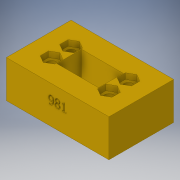
# Autodesk Inventor part: CapForCanBusConnector
Saved by Autodesk Inventor 2018.1 (Build 221171000, 171)
## iProperties
Created: 2017-10-25
Part Number: CapForCanBusConnector
Material: Generic
Document SubType Name: Modeling
Designer: steele
Density: 1 g/cm^3
Appearance: Gold
Author: steele
Autodesk Inventor part; units mm, degrees
note: some values were not read from the file. Chosen so that the rebuilt part matches the saved one: direction of "Emboss1".
ref_plane "YZ Plane" through (0, 0, 0) normal (1, 0, 0) x (0, 1, 0)
ref_plane "XZ Plane" through (0, 0, 0) normal (0, 1, 0) x (-1, 0, 0)
ref_plane "XY Plane" through (0, 0, 0) normal (0, 0, 1) x (1, 0, 0)
sketch "Sketch1" plane through (0, 0, 0) normal (0, 1, 0) x (-1, 0, 0)
  line L0 (18.6817, 11.7856) -> (-18.6817, 11.7856)
  line L1 (-18.6817, 11.7856) -> (-18.6817, -11.7856)
  line L2 (-18.6817, -11.7856) -> (18.6817, -11.7856)
  line L3 (18.6817, -11.7856) -> (18.6817, 11.7856)
  line L4 (18.6817, 11.7856) -> (-18.6817, -11.7856) construction
  line L5 (-18.6817, 11.7856) -> (18.6817, -11.7856) construction
  point P0 (0, 0)
  dimension "d0" = 37.3634
  dimension "d1" = 23.5712
  constraints: 12 end point, 2 midpoint, 2 parallel, 1 horizontal, 1 perpendicular
  measures "d0" distance of L1.end L2.end
  measures "d1" distance of L2.end L0.start
extrude "Extrusion1" add sketch "Sketch1" along normal blind 13.589
sketch "Sketch5" plane through (0, 0, 0) normal (0, -1, 0) x (1, 0, 0)
  line L0 (7.6073, 4.5085) -> (-7.6073, 4.5085)
  line L1 (-7.6073, 4.5085) -> (-7.6073, -4.5085)
  line L2 (-7.6073, -4.5085) -> (7.6073, -4.5085)
  line L3 (7.6073, -4.5085) -> (7.6073, 4.5085)
  line L4 (7.6073, 4.5085) -> (-7.6073, -4.5085) construction
  line L5 (-7.6073, 4.5085) -> (7.6073, -4.5085) construction
  point P0 (0, 0)
  dimension "d25" = 15.2146
  dimension "d26" = 9.017
  constraints: 12 end point, 2 midpoint, 2 parallel, 1 horizontal, 1 perpendicular
  measures "d25" distance of L1.end L2.end
  measures "d26" distance of L2.end L0.start
extrude "Extrusion3" cut sketch "Sketch5" against normal through all
sketch "Sketch8" plane through (0, 13.589, 0) normal (0, 1, 0) x (1, 0, 0)
  circle A0 centre (-10.4521, 3.556) radius 1.632 projected
  line L0 (-7.8168, 5.0775) -> (-7.8168, 2.0345)
  line L1 (-7.8168, 2.0345) -> (-10.4521, 0.5131)
  line L2 (-10.4521, 0.5131) -> (-13.0873, 2.0345)
  line L3 (-13.0873, 2.0345) -> (-13.0873, 5.0775)
  line L4 (-13.0873, 5.0775) -> (-10.4521, 6.5989)
  line L5 (-10.4521, 6.5989) -> (-7.8168, 5.0775)
  circle A1 centre (-10.4521, -3.556) radius 1.632 projected
  line L6 (-7.8169, -2.0345) -> (-7.8169, -5.0775)
  line L7 (-7.8169, -5.0775) -> (-10.4521, -6.5989)
  line L8 (-10.4521, -6.5989) -> (-13.0874, -5.0775)
  line L9 (-13.0874, -5.0775) -> (-13.0874, -2.0345)
  line L10 (-13.0874, -2.0345) -> (-10.4521, -0.5131)
  line L11 (-10.4521, -0.5131) -> (-7.8169, -2.0345)
  circle A2 centre (10.4521, -3.556) radius 1.632 projected
  line L12 (10.4521, -0.5131) -> (13.0873, -2.0345)
  line L13 (13.0873, -2.0345) -> (13.0873, -5.0775)
  line L14 (13.0873, -5.0775) -> (10.4521, -6.5989)
  line L15 (10.4521, -6.5989) -> (7.8168, -5.0775)
  line L16 (7.8168, -5.0775) -> (7.8168, -2.0345)
  line L17 (7.8168, -2.0345) -> (10.4521, -0.5131)
  circle A3 centre (10.4521, 3.556) radius 1.632 projected
  line L18 (13.0874, 5.0775) -> (13.0874, 2.0345)
  line L19 (13.0874, 2.0345) -> (10.4521, 0.5131)
  line L20 (10.4521, 0.5131) -> (7.8169, 2.0345)
  line L21 (7.8169, 2.0345) -> (7.8169, 5.0775)
  line L22 (7.8169, 5.0775) -> (10.4521, 6.5989)
  line L23 (10.4521, 6.5989) -> (13.0874, 5.0775)
  line L24 (18.6817, 11.7856) -> (-18.6817, 11.7856) construction
  line L25 (0, 11.7856) -> (0, -11.7856) construction
  line L26 (-18.6817, -11.7856) -> (18.6817, -11.7856) construction
  point P0 (0, 0)
  dimension "d43" = 5.2705
  constraints: 50 end point, 4 coincident, 4 parallel, 3 equal length, 2 midpoint, 52 other
  measures "d43" distance between parallel lines of L1 L4
extrude "Extrusion5" cut sketch "Sketch8" against normal blind 2.0955 contours A0 | L0 L1 L2 L3 L4 L5 | A1 | L6 L7 L8 L9 L10 L11 | A2 | L12 L13 L14 L15 L16 L17 | A3 | L18 L19 L20 L21 L22 L23
sketch "Sketch13" plane through (0, 11.4935, 0) normal (0, 1, 0) x (1, 0, 0)
  line L0 (-10.4521, 6.5989) -> (-7.8168, 5.0775) construction
  line L1 (-7.8169, -5.0775) -> (-10.4521, -6.5989) construction
  line L2 (-10.4521, 6.5989) -> (-10.4521, -6.5989) construction
  line L3 (10.4521, 6.5989) -> (13.0874, 5.0775) construction
  line L4 (10.4521, -6.5989) -> (7.8168, -5.0775) construction
  line L5 (10.4521, 6.5989) -> (10.4521, -6.5989) construction
  line L6 (-13.0873, 2.0345) -> (-13.0873, 5.0775) construction
  line L7 (-13.0873, 3.556) -> (13.0874, 3.556) construction
  line L8 (13.0874, 5.0775) -> (13.0874, 2.0345) construction
  line L9 (-13.0874, -5.0775) -> (-13.0874, -2.0345) construction
  line L10 (-13.0874, -3.556) -> (13.0873, -3.556) construction
  line L11 (13.0873, -2.0345) -> (13.0873, -5.0775) construction
  point P0 (0, 0)
  point P1 (-10.4521, 3.556)
  point P2 (10.4521, 3.556)
  point P3 (10.4521, -3.556)
  point P4 (-10.4521, -3.556)
  constraints: 8 end point, 8 point on line, 4 midpoint, 2 vertical
hole "Hole9" at (-10.4521, 11.4935, -3.556) at (10.4521, 11.4935, -3.556) at (10.4521, 11.4935, 3.556) at (-10.4521, 11.4935, 3.556) direction (0, -1, 0) diameter 3.302 end through all
sketch "Sketch17" plane through (-18.6817, 0, 11.7856) normal (0, 0, 1) x (1, 0, 0)
  line L0 (0, 0) -> (0, 13.589) construction
  line L1 (0, 6.7945) -> (37.3634, 6.7945) construction
  line L2 (37.3634, 0) -> (37.3634, 13.589) construction
  spline S0 degree 2 poles (15.3892, 8.852) (15.3892, 9.0867) (15.5423, 9.4769) (15.6757, 9.6177) knots 0 0 0 1 2 2 2
  spline S1 degree 2 poles (15.6757, 9.6177) (15.8017, 9.7536) (16.1697, 9.9043) (16.3574, 9.9043) knots 0 0 0 1 2 2 2
  spline S2 degree 2 poles (16.3574, 9.9043) (16.5674, 9.9043) (16.9082, 9.7635) (17.0342, 9.6301) knots 0 0 0 1 2 2 2
  spline S3 degree 2 poles (17.0342, 9.6301) (17.1923, 9.4621) (17.3652, 8.9187) (17.3652, 8.5013) knots 0 0 0 1 2 2 2
  spline S4 degree 2 poles (17.3652, 8.5013) (17.3652, 8.1234) (17.1948, 7.4466) (17.0293, 7.2218) knots 0 0 0 1 2 2 2
  spline S5 degree 2 poles (17.0293, 7.2218) (16.8539, 6.9847) (16.3599, 6.7352) (15.9993, 6.7352) knots 0 0 0 1 2 2 2
  spline S6 degree 2 poles (15.9993, 6.7352) (15.9178, 6.7352) (15.7325, 6.7525) (15.6535, 6.7772) knots 0 0 0 1 2 2 2
  line L3 (15.6535, 6.7772) -> (15.6535, 7.1699)
  line L4 (15.6535, 7.1699) -> (15.6732, 7.1699)
  spline S7 degree 2 poles (15.6732, 7.1699) (15.7251, 7.1403) (15.9425, 7.0884) (16.0536, 7.0884) knots 0 0 0 1 2 2 2
  spline S8 degree 2 poles (16.0536, 7.0884) (16.4537, 7.0884) (16.9107, 7.617) (16.9428, 8.1061) knots 0 0 0 1 2 2 2
  spline S9 degree 2 poles (16.9428, 8.1061) (16.7798, 7.9949) (16.4834, 7.8937) (16.308, 7.8937) knots 0 0 0 1 2 2 2
  spline S10 degree 2 poles (16.308, 7.8937) (16.1401, 7.8937) (15.8609, 7.9678) (15.7202, 8.074) knots 0 0 0 1 2 2 2
  spline S11 degree 2 poles (15.7202, 8.074) (15.5571, 8.1999) (15.3892, 8.5828) (15.3892, 8.852) knots 0 0 0 1 2 2 2
  spline S12 degree 2 poles (16.9527, 8.5927) (16.9527, 8.9014) (16.8391, 9.2917) (16.7378, 9.3979) knots 0 0 0 1 2 2 2
  spline S13 degree 2 poles (16.7378, 9.3979) (16.6489, 9.4967) (16.4636, 9.5708) (16.3549, 9.5708) knots 0 0 0 1 2 2 2
  spline S14 degree 2 poles (16.3549, 9.5708) (16.103, 9.5708) (15.8041, 9.2102) (15.8041, 8.8693) knots 0 0 0 1 2 2 2
  spline S15 degree 2 poles (15.8041, 8.8693) (15.8041, 8.6767) (15.9029, 8.4272) (16.0116, 8.3383) knots 0 0 0 1 2 2 2
  spline S16 degree 2 poles (16.0116, 8.3383) (16.0907, 8.274) (16.2858, 8.232) (16.3994, 8.232) knots 0 0 0 1 2 2 2
  spline S17 degree 2 poles (16.3994, 8.232) (16.5303, 8.232) (16.8317, 8.3234) (16.9453, 8.4) knots 0 0 0 1 2 2 2
  spline S18 degree 2 poles (16.9453, 8.4) (16.9477, 8.4297) (16.9527, 8.5309) (16.9527, 8.5927) knots 0 0 0 1 2 2 2
  spline S19 degree 2 poles (18.6817, 6.7253) (18.4545, 6.7253) (18.0815, 6.8612) (17.9506, 6.9872) knots 0 0 0 1 2 2 2
  spline S20 degree 2 poles (17.9506, 6.9872) (17.8221, 7.1107) (17.6888, 7.4466) (17.6888, 7.6368) knots 0 0 0 1 2 2 2
  spline S21 degree 2 poles (17.6888, 7.6368) (17.6888, 7.8838) (17.953, 8.2987) (18.205, 8.4222) knots 0 0 0 1 2 2 2
  line L5 (18.205, 8.4222) -> (18.205, 8.4346)
  spline S22 degree 2 poles (18.205, 8.4346) (17.9802, 8.5655) (17.7629, 8.8767) (17.7629, 9.1089) knots 0 0 0 1 2 2 2
  spline S23 degree 2 poles (17.7629, 9.1089) (17.7629, 9.4522) (18.2816, 9.9117) (18.6817, 9.9117) knots 0 0 0 1 2 2 2
  spline S24 degree 2 poles (18.6817, 9.9117) (19.0967, 9.9117) (19.5981, 9.4769) (19.5981, 9.1361) knots 0 0 0 1 2 2 2
  spline S25 degree 2 poles (19.5981, 9.1361) (19.5981, 8.9311) (19.3585, 8.5309) (19.1337, 8.4173) knots 0 0 0 1 2 2 2
  line L6 (19.1337, 8.4173) -> (19.1337, 8.405)
  spline S26 degree 2 poles (19.1337, 8.405) (19.4005, 8.2814) (19.6746, 7.9258) (19.6746, 7.6442) knots 0 0 0 1 2 2 2
  spline S27 degree 2 poles (19.6746, 7.6442) (19.6746, 7.2539) (19.1065, 6.7253) (18.6817, 6.7253) knots 0 0 0 1 2 2 2
  spline S28 degree 2 poles (19.2547, 7.6047) (19.2547, 7.7924) (19.1065, 8.0147) (18.8966, 8.1283) knots 0 0 0 1 2 2 2
  spline S29 degree 2 poles (18.8966, 8.1283) (18.8274, 8.1678) (18.5952, 8.2592) (18.4495, 8.3185) knots 0 0 0 1 2 2 2
  spline S30 degree 2 poles (18.4495, 8.3185) (18.2816, 8.2073) (18.1012, 7.8764) (18.1012, 7.6664) knots 0 0 0 1 2 2 2
  spline S31 degree 2 poles (18.1012, 7.6664) (18.1012, 7.3898) (18.4347, 7.0292) (18.6866, 7.0292) knots 0 0 0 1 2 2 2
  spline S32 degree 2 poles (18.6866, 7.0292) (18.9435, 7.0292) (19.2547, 7.3379) (19.2547, 7.6047) knots 0 0 0 1 2 2 2
  spline S33 degree 2 poles (19.1979, 9.1311) (19.1979, 9.3361) (18.9238, 9.6103) (18.6792, 9.6103) knots 0 0 0 1 2 2 2
  spline S34 degree 2 poles (18.6792, 9.6103) (18.4569, 9.6103) (18.1729, 9.3658) (18.1729, 9.1558) knots 0 0 0 1 2 2 2
  spline S35 degree 2 poles (18.1729, 9.1558) (18.1729, 9.0052) (18.3186, 8.7952) (18.4643, 8.7112) knots 0 0 0 1 2 2 2
  spline S36 degree 2 poles (18.4643, 8.7112) (18.5261, 8.6767) (18.7879, 8.5556) (18.8941, 8.521) knots 0 0 0 1 2 2 2
  spline S37 degree 2 poles (18.8941, 8.521) (19.072, 8.6569) (19.1979, 8.9459) (19.1979, 9.1311) knots 0 0 0 1 2 2 2
  line L7 (21.7742, 6.7945) -> (20.2872, 6.7945)
  line L8 (20.2872, 6.7945) -> (20.2872, 7.1057)
  line L9 (20.2872, 7.1057) -> (20.8405, 7.1057)
  line L10 (20.8405, 7.1057) -> (20.8405, 9.1484)
  line L11 (20.8405, 9.1484) -> (20.2872, 9.1484)
  line L12 (20.2872, 9.1484) -> (20.2872, 9.4275)
  spline S38 degree 2 poles (20.2872, 9.4275) (20.6009, 9.4275) (20.8973, 9.6054) (20.9171, 9.8524) knots 0 0 0 1 2 2 2
  line L13 (20.9171, 9.8524) -> (21.2332, 9.8524)
  line L14 (21.2332, 9.8524) -> (21.2332, 7.1057)
  line L15 (21.2332, 7.1057) -> (21.7742, 7.1057)
  line L16 (21.7742, 7.1057) -> (21.7742, 6.7945)
  point P0 (18.6817, 0)
  constraints: 2 end point, 2 midpoint, 1 horizontal
emboss "Emboss1" sketch "Sketch17" operation cut depth 2.54 direction (0, 0, -1)
equation "\"d0\" = PartWidth"
equation "\"d1\" = PartLength"
equation "\"d2\" = capHeight"
equation "\"d25\" = canWireHolderWidth + boardGap"
equation "\"d26\" = canWireHolderLength + boardGap"
equation "\"d43\" = hexNutWidth"
equation "\"d46\" = hexNutHeight"
equation "\"d76\" = boltHoleDiam"
equation "\"HoleWidth\" = 20.9042"
equation "\"HoleLength\" = 7.112"
equation "\"BaseOffset\" = 5.08"
equation "\"PartWidth\" = CanBaseWidth + 2 * BaseOffset"
equation "\"PartLength\" = CanBaseLength + 2 * BaseOffset"
equation "\"boardGap\" = 0.508"
equation "\"boltHeadHeight\" = 3.175"
equation "\"boltHeadDiam\" = 5.08"
equation "\"capHeight\" = 13.589"
equation "\"canWireHolderWidth\" = 14.7066"
equation "\"canWireHolderLength\" = 8.509"
equation "\"hexNutWidth\" = 5.2705"
equation "\"hexNutHeight\" = 2.0955"
equation "\"boltHoleDiam\" = 3.302"
equation "\"CanBaseWidth\" = 27.2034"
equation "\"CanBaseLength\" = 13.4112"
body "Solid1"
